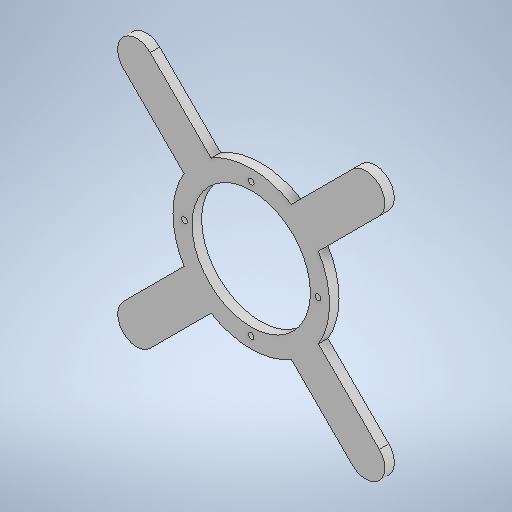
# Autodesk Inventor part: Base
Saved by Autodesk Inventor 2025.1 (Build 291241020, 241B)
## iProperties
Created: 2024-09-22
Part Number: Base
Material: 일반
Document SubType Name: Modeling
Designer: daare
Density: 1 g/cm^3
Appearance: 기본값
Author: daare
Autodesk Inventor part; units mm, degrees
ref_plane "YZ Plane" through (0, 0, 0) normal (1, 0, 0) x (0, 1, 0)
ref_plane "XZ Plane" through (0, 0, 0) normal (0, 1, 0) x (-1, 0, 0)
ref_plane "XY Plane" through (0, 0, 0) normal (0, 0, 1) x (1, 0, 0)
sketch "스케치1" plane through (0, 0, 0) normal (0, 0, 1) x (1, 0, 0)
  arc A0 (-52.9289, 67.0711) -> (-67.0711, 52.9289) centre (-60, 60) ccw
  line L0 (-67.0711, 52.9289) -> (-28.2843, 14.1421)
  line L1 (-52.9289, 67.0711) -> (-14.1421, 28.2843)
  line L2 (-60, 60) -> (0, 0)
  arc A1 (-27.8247, 13.6671) -> (-28.2843, 14.1421) centre (-42.4264, 0) ccw
  line L3 (-89.2706, 0) -> (16.6284, 0) projected
  arc A2 (-14.1421, 28.2843) -> (-13.6671, 27.8247) centre (0, 42.4264) ccw
  line L4 (0, -16.6284) -> (0, 89.2706) projected
  line L5 (-40, 0) -> (-30, 0)
  circle A3 centre (-35, 0) radius 1.5
  circle A4 centre (0, 35) radius 1.5
  arc A5 (0, 31) -> (-31, 0) centre (0, 0) ccw
  arc A6 (0, 41) -> (-41, 0) centre (0, 0) ccw
  point P0 (-22.4264, 0)
  point P1 (0, 22.4264)
  point P2 (-47.1079, 32.9658)
  point P3 (-31.7366, 17.5944)
  point P4 (-32.9658, 47.1079)
  point P5 (-17.5944, 31.7366)
  point P6 (-36.5, 0)
  point P7 (-33.5, 0)
  point P8 (0, 33.5)
  point P9 (0, 36.5)
  point P10 (-21.0448, 35.1869)
  point P11 (-35.1869, 21.0448)
  dimension "d0" = 60
  dimension "d1" = 60
  dimension "d2" = 20
  dimension "d3" = 20
  dimension "d30" = 35
  dimension "d32" = 3
  dimension "d33" = 62
  dimension "d34" = 10
  constraints: 12 point on circle, 8 end point, 8 point on line, 7 centre point, 6 symmetric about line, 3 tangent, 2 coincident, 2 horizontal alignment, 2 parallel, 1 midpoint, 2 other
  measures "d0" horizontal distance of L2.end L2.start
  measures "d1" horizontal distance of L2.end L2.start
  measures "d2" diameter of A0
  measures "d3" radius of A1
  measures "d30" distance of L2.end point (-35, 0)
  measures "d32" diameter of A3
  measures "d33" diameter of A5
  measures "d34" radial gap between concentric circles of A5 A6
extrude "돌출1" add sketch "스케치1" along normal blind 5 contours L1 A6 L0 A0 | A6 L4 A4 A5 A2 L1 | L1 A2 A5 L2 A6 | A6 L2 A5 A1 L0 | L0 A1 A5 L3 A3 A6
pattern_circular "원형 패턴1" count 4 over 360 about axis through (0, 0, -10) along (0, 0, 1) of "돌출1"
